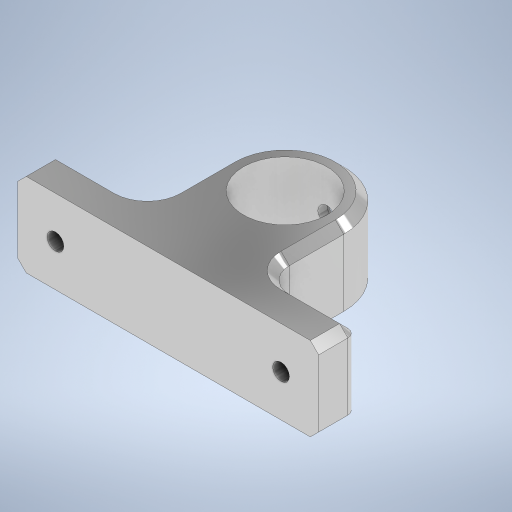
# Autodesk Inventor part: pt2
Saved by Autodesk Inventor 2024.2 (Build 282272000, 272)
## iProperties
Created: 2024-10-24
Part Number: pt2
Material: Generic
Document SubType Name: Modeling
Designer: Precisión-05
Density: 1 g/cm^3
Appearance: Chrome - Polished
Author: Precisión-05
Autodesk Inventor part; units mm, degrees
ref_plane "YZ Plane" through (0, 0, 0) normal (1, 0, 0) x (0, 1, 0)
ref_plane "XY Plane" through (0, 0, 0) normal (0, 0, 1) x (1, 0, 0)
sketch "Sketch1" plane through (0, 0, 0) normal (0, 0, 1) x (1, 0, 0)
  circle A0 centre (0, 0) radius 5
  circle A1 centre (0, 0) radius 7
  line L0 (-18, -9.5) -> (-10, -9.5)
  line L1 (18, -9.5) -> (10, -9.5)
  line L2 (0, -14) -> (18, -14)
  line L3 (0, -14) -> (-18, -14)
  line L4 (-7, 0) -> (-7, -9.5)
  line L5 (-7, -9.5) -> (-18, -9.5)
  line L6 (-18, -9.5) -> (-18, -14)
  line L7 (-18, -14) -> (18, -14)
  line L8 (18, -14) -> (18, -9.5)
  line L9 (18, -9.5) -> (7, -9.5)
  line L10 (7, -9.5) -> (7, 0)
  point P0 (-10.8595, -8.0551)
  dimension "d0" = 14
  dimension "d1" = 10
  dimension "d2" = 4.5
  dimension "d3" = 0
  dimension "d4" = 11
  dimension "d5" = 36
  dimension "d6" = 9.5
  dimension "d7" = 8
  dimension "d8" = 18
  dimension "d9" = 28
  dimension "d10" = 1.4449
  dimension "d11" = 28.8595
  constraints: 18 end point, 3 perpendicular, 2 centre point, 2 coincident, 2 horizontal, 2 point on circle, 2 tangent, 1 collinear, 1 parallel, 1 point on line, 1 vertical, 6 other
  measures "d0" diameter of A1
  measures "d1" diameter of A0
  measures "d2" distance between parallel lines of L7 L9
  measures "d3" distance between parallel lines of L9 L5
  measures "d4" distance between parallel lines of L8 L10
  measures "d5" distance between parallel lines of L8 L6
  measures "d6" distance from line of point (0, 0) L1
  measures "d7" distance from line of L1.end L8
  measures "d8" distance from line of point (0, -14) L8
  measures "d9" distance from line of L0.end L8
  measures "d10" distance from line of point (-10.859, -8.055) L9
  measures "d11" distance from line of point (-10.859, -8.055) L8
extrude "Extrusion1" add sketch "Sketch1" along normal blind 10
fillet "Fillet1" radius 1 2 edges at (18, -9.5, 5) (-18, -9.5, 5)
fillet "Fillet2" radius 3 2 edges at (7, -9.5, 5) (-7, -9.5, 5)
chamfer "Chamfer1" distance 1 angle 45 22 edges at (0, 7, 10) (-7, -3.2502, 10) (-9.9998, -9.5, 10) (-13.5, -9.5, 10) (-17.7071, -9.7929, 10) (-18, -12.25, 10) (7, -3.2503, 10) (9.9997, -9.5, 10) (13.5, -9.5, 10) (17.7071, -9.7929, 10) (18, -12.25, 10) (0, 7, 0) (-7, -3.2502, 0) (-9.9998, -9.5, 0) (-13.5, -9.5, 0) (-17.7071, -9.7929, 0) (-18, -12.25, 0) (7, -3.2503, 0) (9.9997, -9.5, 0) (13.5, -9.5, 0) (17.7071, -9.7929, 0) (18, -12.25, 0)
sketch "Sketch2" plane through (10, -9.5, 1) normal (0, 1, 0) x (1, 0, 0)
  line L0 (-27, 0) -> (-20, 0) projected
  line L1 (-27, -8) -> (-27, 0) projected
  line L2 (-20, -8) -> (-27, -8) projected
  line L3 (-20, 0) -> (-20, -8) projected
  line L4 (0, 0) -> (7, 0) projected
  line L5 (0, -8) -> (0, 0) projected
  line L6 (7, -8) -> (0, -8) projected
  line L7 (7, 0) -> (7, -8) projected
  line L8 (-27, -8) -> (-20, -8)
  line L9 (-20, -8) -> (-20, 0)
  line L10 (-20, 0) -> (-27, 0)
  line L11 (-27, 0) -> (-27, -8)
  line L12 (-27, -8) -> (-20, 0) construction
  line L13 (-20, -8) -> (-27, 0) construction
  line L14 (0, -8) -> (7, -8)
  line L15 (7, -8) -> (7, 0)
  line L16 (7, 0) -> (0, 0)
  line L17 (0, 0) -> (0, -8)
  line L18 (0, -8) -> (7, 0) construction
  line L19 (7, -8) -> (0, 0) construction
  point P0 (-10, 1)
  point P1 (-23.5, -4)
  point P2 (3.5, -4)
  point P3 (-23.5, -4)
  point P4 (3.5, -4)
  constraints: 24 end point, 4 midpoint, 4 parallel, 2 coincident, 2 horizontal, 2 perpendicular
hole "Hole1" at (-13.5, -9.5, 5) at (13.5, -9.5, 5) direction (0, -1, 0) diameter 2 end through all
ref_plane "Work Plane1" through (0, 7, 0) normal (0, 1, 0) x (-1, 0, 0)
sketch "Sketch3" plane through (0, 7, 0) normal (0, 1, 0) x (-1, 0, 0)
  line L0 (7, 1) -> (-7, 1) projected
  line L1 (7, 1) -> (7, 9) projected
  line L2 (-7, 9) -> (7, 9) projected
  line L3 (-7, 1) -> (-7, 9) projected
  line L4 (7, 9) -> (-7, 9)
  line L5 (-7, 9) -> (-7, 1)
  line L6 (-7, 1) -> (7, 1)
  line L7 (7, 1) -> (7, 9)
  line L8 (7, 9) -> (-7, 1) construction
  line L9 (-7, 9) -> (7, 1) construction
  point P0 (0, 0)
  point P1 (0, 5)
  point P2 (0, 5)
  constraints: 12 end point, 2 midpoint, 2 parallel, 1 coincident, 1 horizontal, 1 perpendicular
hole "Hole2" at (0, 7, 5) direction (0, -1, 0) diameter 2 depth 8 tip angle 118 countersink diameter 4 countersink angle 90
body "Solid1"
